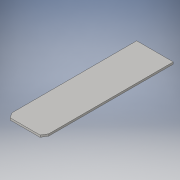
# Autodesk Inventor part: Control Board
Saved by Autodesk Inventor 2016 (Build 200138000, 138)
## iProperties
Created: 2017-09-15
Part Number: Control Board
Material: Generic
Document SubType Name: Modeling
Designer: Student
Density: 1 g/cm^3
Appearance: Default
Author: Student
Autodesk Inventor part; units mm, degrees
ref_plane "YZ Plane" through (0, 0, 0) normal (1, 0, 0) x (0, 1, 0)
ref_plane "XZ Plane" through (0, 0, 0) normal (0, 1, 0) x (-1, 0, 0)
ref_plane "XY Plane" through (0, 0, 0) normal (0, 0, 1) x (1, 0, 0)
sketch "Sketch1" plane through (0, 0, 0) normal (0, 1, 0) x (-1, 0, 0)
  line L0 (47.9603, 101.1149) -> (-52.1157, 101.1149)
  line L1 (-52.1157, 101.1149) -> (-52.1157, -254.4851)
  line L2 (-52.1157, -254.4851) -> (47.9603, -254.4851)
  line L3 (47.9603, -254.4851) -> (47.9603, 101.1149)
  point P0 (0, 0)
  dimension "d0" = 100.076
  dimension "d1" = 355.6
  constraints: 8 end point, 2 parallel, 1 horizontal, 1 perpendicular
  measures "d0" distance of L0.start L0.end
  measures "d1" distance of L2.end L0.start
extrude "Extrusion1" add sketch "Sketch1" along normal blind 5.4102
sketch "Sketch4" plane through (0, 5.4102, 0) normal (0, 1, 0) x (1, 0, 0)
  line L0 (-47.9603, 254.4851) -> (-47.9603, -101.1149) projected
  line L1 (-47.9603, -86.3829) -> (52.1157, -86.3829)
  line L2 (52.1157, -101.1149) -> (52.1157, 254.4851) projected
  line L3 (-47.9603, -101.1149) -> (52.1157, -101.1149) projected
  line L4 (-47.9603, -101.1149) -> (-38.9433, -101.1149)
  line L5 (-38.9433, -101.1149) -> (-47.9603, -86.3829)
  line L6 (-47.9603, -86.3829) -> (-47.9603, -101.1149)
  line L7 (2.0777, -101.1149) -> (2.0777, -39.9393)
  line L8 (43.0987, -101.1149) -> (52.1157, -86.3829)
  line L9 (43.0987, -101.1149) -> (52.1157, -101.1149)
  line L10 (52.1157, -86.3829) -> (52.1157, -101.1149)
  point P0 (0, 0)
  dimension "d4" = 14.732
  dimension "d5" = 9.017
  constraints: 16 end point, 3 point on line, 2 collinear, 1 horizontal, 1 midpoint, 1 perpendicular, 1 symmetric about line, 1 vertical
  measures "d4" distance between parallel lines of L3 L1
  measures "d5" distance of L0.end L4.end
extrude "Extrusion2" cut sketch "Sketch4" against normal blind 5.4102 contours L5 L3 L0 | L2 L3 L8
body "Solid1"
